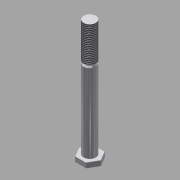
# Autodesk Inventor part: CIM Mount Bolt
Saved by Autodesk Inventor 2013 (Build 170138000, 138)
## iProperties
Created: 2013-01-18
Part Number: CIM Mount Bolt
Material: Aluminum 6061-AHC
Document SubType Name: Modeling
Designer: Naphat
Density: 1 g/cm^3
Author: Naphat
Autodesk Inventor part; units mm, degrees
ref_plane "YZ Plane" through (0, 0, 0) normal (1, 0, 0) x (0, 1, 0)
ref_plane "XZ Plane" through (0, 0, 0) normal (0, 1, 0) x (-1, 0, 0)
ref_plane "XY Plane" through (0, 0, 0) normal (0, 0, 1) x (1, 0, 0)
sketch "Sketch1" plane through (0, 0, 0) normal (0, 1, 0) x (-1, 0, 0)
  circle A0 centre (0, 0) radius 12.7
  dimension "d0" = 25.4
  constraints: 1 centre point, 1 coincident
  measures "d0" diameter of A0
extrude "Extrusion1" add sketch "Sketch1" along normal blind 165.1
sketch "Sketch2" plane through (0, 165.1, 0) normal (0, 1, 0) x (1, 0, 0)
  circle A0 centre (0, 0) radius 12.7 projected
chamfer "Chamfer1" distance 2.54 angle 45 1 edges at (12.7, 165.1, 0)
extrude "Extrusion2" add sketch "Sketch2" along normal blind 76.2
thread "Thread2" size "1-8 UNC" class "2A" standard "ANSI Unified Screw Threads" full length
chamfer "Chamfer2" distance 2.54 angle 45 1 edges at (-12.7, 165.1, 0)
sketch "Sketch3" plane through (0, 0, 0) normal (0, -1, 0) x (1, 0, 0)
  line L0 (0, 20.32) -> (0, -20.32) construction
  line L1 (0, -20.32) -> (11.43, -20.32) construction
  line L2 (11.43, -20.32) -> (-11.43, -20.32)
  line L3 (-11.43, -20.32) -> (-22.86, -0.5227)
  line L4 (-22.86, -0.5227) -> (-11.43, 19.2747)
  line L5 (-11.43, 19.2747) -> (11.43, 19.2747)
  line L6 (11.43, 19.2747) -> (22.86, -0.5227)
  line L7 (22.86, -0.5227) -> (11.43, -20.32)
  point P0 (0, 0)
  dimension "d18" = 20.32
  dimension "d19" = 40.64
  dimension "d20" = 11.43
  dimension "d21" = 22.86
  dimension "d22" = 22.86
  dimension "d23" = 120
  dimension "d24" = 22.86
  dimension "d25" = 22.86
  dimension "d26" = 120
  constraints: 16 end point, 2 parallel, 2 perpendicular, 1 point on line
  measures "d18" distance of point (0, 0) L0.start
  measures "d19" distance of L0.start L0.end
  measures "d20" distance of L0.end L1.end
  measures "d21" distance of L1.end L2.end
  measures "d22" distance of L2.end L3.end
  measures "d23" angle of L2 L3
  measures "d24" distance of L3.end L4.end
  measures "d25" distance of L5.end L6.end
  measures "d26" angle of L5 L6
extrude "Extrusion3" add sketch "Sketch3" along normal blind 12.7
chamfer "Chamfer3" distance 2.54 angle 45 6 edges at (0, -12.7, -20.32) (-17.145, -12.7, -10.4213) (-17.145, -12.7, 9.376) (0, -12.7, 19.2747) (17.145, -12.7, 9.376) (17.145, -12.7, -10.4213)
fillet "Fillet1" radius 1 12 edges at (-10.6968, -11.43, -19.05) (10.6968, -11.43, -19.05) (21.3935, -11.43, -0.5227) (10.6968, -11.43, 18.0047) (-10.6968, -11.43, 18.0047) (-21.3935, -11.43, -0.5227) (-14.9453, -12.7, -9.1513) (-14.9453, -12.7, 8.106) (0, -12.7, 16.7347) (14.9453, -12.7, 8.106) (14.9453, -12.7, -9.1513) (0, -12.7, -17.78)
fillet "Fillet2" radius 1 12 edges at (11.43, -5.0343, -20.32) (22.86, -5.0343, -0.5227) (11.43, -5.0343, 19.2747) (-11.43, -5.0343, 19.2747) (-22.86, -5.0343, -0.5227) (-11.43, -5.0343, -20.32) (-17.145, 0, 9.376) (-17.145, 0, -10.4213) (0, 0, 19.2747) (17.145, 0, 9.376) (17.145, 0, -10.4213) (0, 0, -20.32)
body "Solid1"
